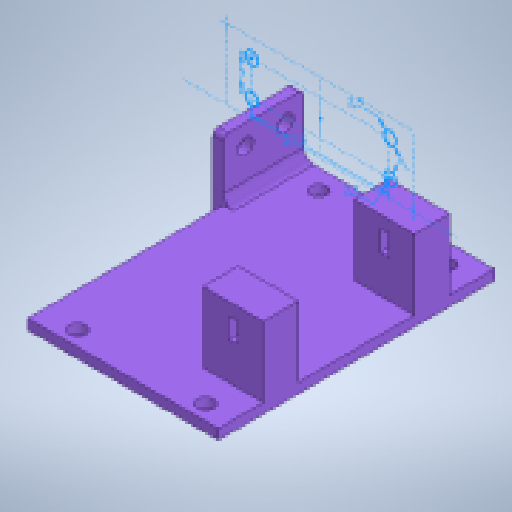
# Autodesk Inventor part: креп_сервы
Saved by Autodesk Inventor 2023.1 (Build 271208000, 208)
## iProperties
Created: 2026-02-03
Part Number: креп_сервы
Material: Типовые
Document SubType Name: Modeling
Designer: DELL
Density: 1 g/cm^3
Appearance: Фиолетовый
Author: DELL
Autodesk Inventor part; units mm, degrees
ref_plane "YZ Plane" through (0, 0, 0) normal (1, 0, 0) x (0, 1, 0)
ref_plane "XZ Plane" through (0, 0, 0) normal (0, 1, 0) x (-1, 0, 0)
ref_plane "XY Plane" through (0, 0, 0) normal (0, 0, 1) x (1, 0, 0)
sketch "Эскиз1" plane through (0, 0, 0) normal (0, 1, 0) x (-1, 0, 0)
  line L0 (-19, 27.5) -> (19, 27.5)
  line L1 (19, 27.5) -> (19, -27.5)
  line L2 (19, -27.5) -> (-19, -27.5)
  line L3 (-19, -27.5) -> (-19, 27.5)
  line L4 (-19, 27.5) -> (19, -27.5) construction
  line L5 (19, 27.5) -> (-19, -27.5) construction
  point P0 (0, 0)
  dimension "d10" = 55
  dimension "d11" = 38
  constraints: 12 end point, 2 midpoint, 2 parallel, 1 horizontal, 1 perpendicular
  measures "d10" distance of L0.end L1.end
  measures "d11" distance of L1.end L2.end
extrude "Выдавливание1" add sketch "Эскиз1" along normal blind 2
sketch "Эскиз2" plane through (0, 2, 0) normal (0, 1, 0) x (1, 0, 0)
  line L0 (7, -18.55) -> (19, -18.55)
  line L1 (19, -18.55) -> (19, -11.55)
  line L2 (19, -11.55) -> (7, -11.55)
  line L3 (7, -11.55) -> (7, -18.55)
  line L4 (7, -18.55) -> (19, -11.55) construction
  line L5 (19, -18.55) -> (7, -11.55) construction
  line L6 (7, 11.55) -> (19, 11.55)
  line L7 (19, 11.55) -> (19, 18.55)
  line L8 (19, 18.55) -> (7, 18.55)
  line L9 (7, 18.55) -> (7, 11.55)
  line L10 (7, 11.55) -> (19, 18.55) construction
  line L11 (19, 11.55) -> (7, 18.55) construction
  line L12 (19, -27.5) -> (19, 27.5) projected
  line L13 (-19, 27.5) -> (-19, -27.5) projected
  line L14 (-19, 0) -> (19, 0)
  point P0 (0, 0)
  point P1 (13, -15.05)
  point P2 (13, 15.05)
  point P3 (0, 0)
  dimension "d2" = 12
  dimension "d3" = 7
  dimension "d4" = 12
  dimension "d5" = 7
  dimension "d12" = 0
  dimension "d15" = 0
  dimension "d25" = 11.55
  dimension "d26" = 11.55
  constraints: 26 end point, 7 midpoint, 4 parallel, 2 horizontal, 2 perpendicular
  measures "d2" distance of L1.end L2.end
  measures "d3" distance of L0.end L1.end
  measures "d4" distance of L7.end L8.end
  measures "d5" distance of L6.end L7.end
  measures "d12" distance between parallel lines of L12 L1
  measures "d15" distance between parallel lines of L12 L7
  measures "d25" distance from line of L6 point (0, 0)
  measures "d26" distance between parallel lines of L14 L2
extrude "Выдавливание2" add sketch "Эскиз2" along normal blind 14
sketch "Эскиз4" plane through (0, 2, 0) normal (0, 1, 0) x (1, 0, 0)
  circle A0 centre (15, 7.55) radius 1.6
  circle A1 centre (11, -7.55) radius 1.6
  line L0 (19, -27.5) -> (19, 27.5) projected
  line L1 (7, -11.55) -> (7, -18.55) projected
  line L2 (7, 11.55) -> (19, 11.55) projected
  line L3 (19, -11.55) -> (7, -11.55) projected
  point P0 (0, 0)
  dimension "d17" = 3.2
  dimension "d18" = 3.2
  dimension "d19" = 4
  dimension "d20" = 4
  dimension "d21" = 4
  dimension "d22" = 4
  constraints: 2 centre point
  measures "d17" diameter of A0
  measures "d18" diameter of A1
  measures "d19" distance from line of L0 A0.centre
  measures "d20" distance from line of L1 A1.centre
  measures "d21" distance from line of L2 A0.centre
  measures "d22" distance from line of L3 A1.centre
extrude "Выдавливание3" cut sketch "Эскиз4" against normal blind 14
sketch "Эскиз5" plane through (19, 2, 18.55) normal (1, 0, 0) x (0, 0, 1)
  circle A0 centre (-32.3, -3.5) radius 1.25
  circle A1 centre (-32.3, -10.5) radius 1.25
  circle A2 centre (-4.8, -10.5) radius 1.25
  circle A3 centre (-4.8, -3.5) radius 1.25
  line L0 (-4.8, -10.5) -> (-32.3, -10.5) construction
  line L1 (-32.3, -10.5) -> (-32.3, -3.5) construction
  line L2 (-32.3, -3.5) -> (-4.8, -3.5) construction
  line L3 (-4.8, -3.5) -> (-4.8, -10.5) construction
  line L4 (0, 0) -> (0, -14) construction
  line L5 (-37.1, 0) -> (-37.1, -14) construction
  line L6 (0, 0) -> (-37.1, 0) construction
  line L7 (-37.1, 0) -> (-37.1, -14) construction
  line L8 (-37.1, -14) -> (0, -14) construction
  line L9 (0, -14) -> (0, 0) construction
  line L10 (-18.55, -14) -> (-18.55, 0) construction
  line L11 (-46.05, 0) -> (8.95, 0) construction
  line L12 (-18.55, -3.5) -> (-18.55, -10.5) construction
  point P0 (-18.55, -7)
  dimension "d51" = 27.5
  dimension "d52" = 7
  dimension "d55" = 2.5
  dimension "d56" = 2.5
  constraints: 20 end point, 6 midpoint, 4 centre point, 4 parallel, 2 coincident, 2 horizontal, 2 perpendicular
  measures "d51" distance of L1.end L2.end
  measures "d52" distance of L0.end L1.end
  measures "d55" diameter of A3
  measures "d56" diameter of A2
extrude "Выдавливание4" cut sketch "Эскиз5" against normal blind 14
sketch "Эскиз6" plane through (0, 2, 0) normal (0, 1, 0) x (1, 0, 0)
  circle A0 centre (-12, -24.5) radius 1.6
  circle A1 centre (-12, 23.5) radius 1.6
  circle A2 centre (13.5, -24.5) radius 1.6
  circle A3 centre (13.5, 23.5) radius 1.6
  point P0 (0, 0)
  constraints: 4 centre point, 8 other
extrude "Выдавливание5" cut sketch "Эскиз6" against normal blind 10
sketch "Эскиз7" plane through (7, 2, 18.55) normal (0, 0, 1) x (1, 0, 0)
  line L0 (12, 14) -> (0, 14) projected
  line L1 (6, 14) -> (6, -2) construction
  line L2 (12, -2) -> (-26, -2) projected
  line L3 (0, 0) -> (0, 14) projected
  line L4 (0, 7) -> (12, 7) construction
  line L5 (12, 0) -> (12, 14) projected
  line L6 (12, 4.75) -> (12, 2.25) projected
  line L7 (0, 9.5) -> (12, 9.5)
  line L8 (6.8, 7.45) -> (5.2, 7.45)
  line L9 (5.2, 7.45) -> (5.2, 11.55)
  line L10 (5.2, 11.55) -> (6.8, 11.55)
  line L11 (6.8, 11.55) -> (6.8, 7.45)
  line L12 (6.8, 7.45) -> (5.2, 11.55) construction
  line L13 (5.2, 7.45) -> (6.8, 11.55) construction
  point P0 (-7, -2)
  point P1 (0, 8.25)
  point P2 (0, 10.75)
  point P3 (6, 9.5)
  dimension "d31" = 4.5
  dimension "d32" = 1.6
  dimension "d33" = 4.1
  constraints: 18 end point, 6 midpoint, 2 parallel, 2 perpendicular, 2 point on line, 1 horizontal, 1 vertical
  measures "d31" distance between parallel lines of L0 L7
  measures "d32" distance of L9.end L10.end
  measures "d33" distance of L8.end L9.end
extrude "Выдавливание6" cut sketch "Эскиз7" against normal blind 12 contours L11 L8 L9 L7 | L7 L9 L10 L11
mirror "Зеркальное отражение1" about plane through (0, 0, 0) normal (0, 0, 1) of "Выдавливание6"
sketch "Эскиз8" plane through (-19, 0, -27.5) normal (-1, 0, 0) x (0, 0, 1)
  line L0 (0, 0) -> (16, 0)
  line L1 (16, 0) -> (16, 14)
  line L2 (16, 14) -> (0, 14)
  line L3 (0, 14) -> (0, 0)
  point P0 (27.5, 0)
  dimension "d38" = 16
  dimension "d39" = 14
  constraints: 8 end point, 2 parallel, 1 horizontal, 1 perpendicular
  measures "d38" distance of L2.end L1.end
  measures "d39" distance of L1.end L0.end
extrude "Выдавливание7" add sketch "Эскиз8" along normal blind 2
sketch "Эскиз9" plane through (-21, 0, -27.5) normal (-1, 0, 0) x (0, 0, 1)
  line L0 (0, 14) -> (0, 0) construction
  line L1 (0, 10) -> (16, 10) construction
  line L2 (16, 0) -> (16, 14) construction
  line L3 (16, 14) -> (0, 14) construction
  circle A0 centre (3.5886, 10) radius 1.6
  circle A1 centre (11.5886, 10) radius 1.6
  line L4 (3.5886, 10) -> (11.5886, 10)
  line L5 (8, 14) -> (8, 2)
  line L6 (55, 2) -> (0, 2) projected
  point P0 (27.5, 0)
  point P1 (0, 12)
  point P2 (16, 12)
  point P3 (14, 14)
  point P4 (2, 14)
  dimension "d43" = 4
  dimension "d44" = 3.2
  dimension "d45" = 3.2
  dimension "d46" = 8
  constraints: 6 end point, 5 point on line, 2 centre point, 1 collinear, 1 horizontal, 1 midpoint, 1 perpendicular
  measures "d43" distance between parallel lines of L3 L1
  measures "d44" diameter of A0
  measures "d45" diameter of A1
  measures "d46" distance of L4.end L4.start
extrude "Выдавливание8" cut sketch "Эскиз9" against normal blind 2
fillet "Сопряжение2" radius 2 1 edges at (-19, 2, -19.5)
fillet "Сопряжение3" radius 1 2 edges at (-20, 14, -27.5) (-20, 14, -11.5)
